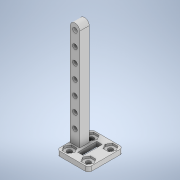
# Autodesk Inventor part: new_stand
Saved by Autodesk Inventor 2020 (Build 240168000, 168)
## iProperties
Created: 2023-05-31
Part Number: new_stand
Material: Типовые
Document SubType Name: Modeling
Designer: denis
Density: 1 g/cm^3
Appearance: По умолчанию
Author: denis
Autodesk Inventor part; units mm, degrees
ref_plane "YZ Plane" through (0, 0, 0) normal (1, 0, 0) x (0, 1, 0)
ref_plane "XZ Plane" through (0, 0, 0) normal (0, 1, 0) x (-1, 0, 0)
ref_plane "XY Plane" through (0, 0, 0) normal (0, 0, 1) x (1, 0, 0)
sketch "Эскиз1" plane through (0, 0, 0) normal (0, 1, 0) x (-1, 0, 0)
  line L0 (-10, 11) -> (10, -11) construction
  line L1 (9.5, 11) -> (-9.5, -11) construction
  line L2 (0, 11) -> (0, -11) construction
  line L3 (9.5, 0) -> (-9.5, 0) construction
  circle A0 centre (6, 7) radius 1.5
  circle A1 centre (6, -7) radius 1.5
  circle A2 centre (-6, 7) radius 1.5
  circle A3 centre (-6, -7) radius 1.5
  line L4 (-1.75, 6) -> (1.75, 6)
  line L5 (1.75, 6) -> (1.75, -6)
  line L6 (1.75, -6) -> (-1.75, -6)
  line L7 (-1.75, -6) -> (-1.75, 6)
  line L8 (-1.75, 6) -> (1.75, -6) construction
  line L9 (1.75, 6) -> (-1.75, -6) construction
  circle A4 centre (6, 7) radius 3.5 construction
  line L10 (7.75, 10.0311) -> (9.5, 7)
  line L11 (9.5, 7) -> (7.75, 3.9689)
  line L12 (7.75, 3.9689) -> (4.25, 3.9689)
  line L13 (4.25, 3.9689) -> (2.5, 7)
  line L14 (2.5, 7) -> (4.25, 10.0311)
  line L15 (4.25, 10.0311) -> (7.75, 10.0311)
  circle A5 centre (6, -7) radius 1.5
  circle A6 centre (6, -7) radius 3.5 construction
  line L16 (7.75, -10.0311) -> (9.5, -7)
  line L17 (9.5, -7) -> (7.75, -3.9689)
  line L18 (7.75, -3.9689) -> (4.25, -3.9689)
  line L19 (4.25, -3.9689) -> (2.5, -7)
  line L20 (2.5, -7) -> (4.25, -10.0311)
  line L21 (4.25, -10.0311) -> (7.75, -10.0311)
  circle A7 centre (-6, 7) radius 1.5
  circle A8 centre (-6, -7) radius 1.5
  circle A9 centre (-6, 7) radius 3.5 construction
  line L22 (-7.75, 10.0311) -> (-9.5, 7)
  line L23 (-9.5, 7) -> (-7.75, 3.9689)
  line L24 (-7.75, 3.9689) -> (-4.25, 3.9689)
  line L25 (-4.25, 3.9689) -> (-2.5, 7)
  line L26 (-2.5, 7) -> (-4.25, 10.0311)
  line L27 (-4.25, 10.0311) -> (-7.75, 10.0311)
  line L28 (-4.25, -3.9689) -> (-2.5, -7)
  line L29 (-7.75, -3.9689) -> (-4.25, -3.9689)
  line L30 (-2.5, -7) -> (-4.25, -10.0311)
  circle A10 centre (-6, -7) radius 1.5
  line L31 (-9.5, -7) -> (-7.75, -3.9689)
  line L32 (-4.25, -10.0311) -> (-7.75, -10.0311)
  circle A11 centre (-6, -7) radius 3.5 construction
  line L33 (-7.75, -10.0311) -> (-9.5, -7)
  line L34 (-8, 11) -> (8, 11)
  line L35 (10, 9) -> (10, -9)
  line L36 (8, -11) -> (-8, -11)
  line L37 (-10, -9) -> (-10, 9)
  line L38 (-10, 11) -> (10, -11) construction
  line L39 (10, 11) -> (-10, -11) construction
  arc A12 (-8, 11) -> (-10, 9) centre (-8, 9) ccw
  arc A13 (10, 9) -> (8, 11) centre (8, 9) ccw
  arc A14 (8, -11) -> (10, -9) centre (8, -9) ccw
  arc A15 (-10, -9) -> (-8, -11) centre (-8, -9) ccw
  line L40 (9.5, 0) -> (6.5, 0) construction
  line L41 (3.5, 3) -> (9.5, 3)
  line L42 (9.5, 3) -> (9.5, -3)
  line L43 (9.5, -3) -> (3.5, -3)
  line L44 (3.5, -3) -> (3.5, 3)
  line L45 (3.5, 3) -> (9.5, -3) construction
  line L46 (9.5, 3) -> (3.5, -3) construction
  point P0 (0, 0)
  point P1 (6, -7)
  point P2 (-6, -7)
  point P3 (-6, -7)
  point P4 (9.5, -3)
  dimension "d5" = 7
  dimension "d0" = 3
  dimension "d1" = 14
  dimension "d2" = 12
  dimension "d3" = 3.5
  dimension "d4" = 12
  dimension "d8" = 360
  dimension "d16" = 20
  dimension "d17" = 22
  dimension "d18" = 2
  dimension "d19" = 2
  dimension "d20" = 3
  dimension "d21" = 6
  dimension "d22" = 6
  constraints: 94 end point, 31 symmetric about line, 12 centre point, 9 parallel, 9 point on line, 8 midpoint, 8 point on circle, 8 tangent, 5 horizontal, 4 coincident, 4 horizontal alignment, 3 perpendicular, 2 equal radius, 2 vertical, 22 other
  measures "d0" diameter of A0
  measures "d1" distance of point (6, -7) A0.centre
  measures "d2" distance of A2.centre A0.centre
  measures "d3" distance of L5.end L6.end
  measures "d4" distance of L4.end L5.end
  measures "d16" distance of L0.end L39.end
  measures "d17" distance of L39.start L0.end
  measures "d18" radius of A12
  measures "d19" radius of A13
  measures "d20" distance of L3.start L40.end
  measures "d21" distance of L42.end L43.end
  measures "d22" distance of L41.end L42.end
extrude "Выдавливание1" add sketch "Эскиз1" along normal blind 70 contours L41 L42 L43 L44
extrude "Выдавливание2" add sketch "Эскиз1" along normal blind 3 contours L34 A13 L35 A14 L36 A15 L37 A12
extrude "Выдавливание3" add sketch "Эскиз1" along normal blind 1.8 contours L10 L11 L12 L13 L14 L15 | L21 L20 L19 L18 L17 L16 | L27 L26 L25 L24 L23 L22 | L28 L30 L32 L33 L31 L29
sketch "Эскиз2" plane through (0, 0, 0) normal (0, 0, 1) x (1, 0, 0)
  line L0 (-9.5, 3) -> (-3.5, 3) projected
  line L1 (-9.5, 3) -> (-3.5, 3)
  line L2 (-3.5, 70) -> (-9.5, 70) projected
  line L3 (-3.5, 3) -> (-3.5, 67)
  line L4 (-6.5, 70) -> (-6.5, 70)
  line L5 (-9.5, 3) -> (-9.5, 70) projected
  line L6 (-9.5, 67) -> (-9.5, 3)
  arc A0 (-3.5, 67) -> (-6.5, 70) centre (-6.5, 67) ccw
  arc A1 (-6.5, 70) -> (-9.5, 67) centre (-6.5, 67) ccw
  circle A2 centre (-6.5, 12) radius 1.5
  circle A3 centre (-6.5, 21) radius 1.5
  circle A4 centre (-6.5, 30) radius 1.5
  circle A5 centre (-6.5, 39) radius 1.5
  circle A6 centre (-6.5, 48) radius 1.5
  circle A7 centre (-6.5, 57) radius 1.5
  circle A8 centre (-6.5, 66) radius 1.5
  line L7 (-9.5, 67) -> (-9.5, 70)
  line L8 (-3.5, 3) -> (-3.5, 70) projected
  line L9 (-3.5, 67) -> (-3.5, 70)
  line L10 (-9.5, 70) -> (-6.5, 70)
  line L11 (-6.5, 70) -> (-3.5, 70)
  point P0 (0, 0)
  dimension "d29" = 3
  dimension "d30" = 3
  dimension "d31" = 9
  dimension "d32" = 3
  dimension "d33" = 3
  dimension "d34" = 3
  dimension "d35" = 3
  dimension "d36" = 3
  dimension "d37" = 3
  dimension "d38" = 9
  dimension "d39" = 9
  dimension "d40" = 9
  dimension "d41" = 9
  dimension "d42" = 9
  dimension "d43" = 9
  constraints: 16 end point, 9 centre point, 7 collinear, 7 tangent, 4 point on circle, 4 point on line, 1 concentric, 1 perpendicular
  measures "d29" radius of A0
  measures "d30" diameter of A2
  measures "d31" distance from line of L0 A2.centre
  measures "d32" diameter of A3
  measures "d33" diameter of A4
  measures "d34" diameter of A5
  measures "d35" diameter of A6
  measures "d36" diameter of A7
  measures "d37" diameter of A8
  measures "d38" distance of A8.centre A7.centre
  measures "d39" distance of A6.centre A7.centre
  measures "d40" distance of A5.centre A6.centre
  measures "d41" distance of A4.centre A5.centre
  measures "d42" distance of A3.centre A4.centre
  measures "d43" distance of A2.centre A3.centre
extrude "Выдавливание4" cut sketch "Эскиз2" along normal mid plane 6 contours L5 A1 A0 L3 L0 | L5 L2 A1 | A0 L2 L8 | A2 | A3 | A4 | A5 | A6 | A7 | A8
extrude "Выдавливание5" add sketch "Эскиз2" along normal mid plane 6 contours L5 A1 A0 L3 L0
